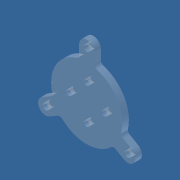
# Autodesk Inventor part: acrylic gripper plate
Saved by Autodesk Inventor 2012 (Build 160160000, 160)
## iProperties
Created: 2012-07-09
Part Number: acrylic gripper plate
Material: Polycarbonate, Clear
Document SubType Name: Modeling
Designer: Ed
Density: 1.2 g/cm^3
Mass: 25.0614 g
Surface Area: 89.5421 cm^2
Volume: 20.8845 cm^3
Author: Ed
Autodesk Inventor part; units mm, degrees
ref_plane "YZ Plane" through (0, 0, 0) normal (1, 0, 0) x (0, 1, 0)
ref_plane "XZ Plane" through (0, 0, 0) normal (0, 1, 0) x (-1, 0, 0)
ref_plane "XY Plane" through (0, 0, 0) normal (0, 0, 1) x (1, 0, 0)
sketch "Sketch1" plane through (0, 0, 0) normal (0, 0, 1) x (1, 0, 0)
  circle A0 centre (0, 0) radius 30
  line L0 (-6.35, 29.3203) -> (6.35, 29.3203)
  line L1 (6.35, 29.3203) -> (6.35, 40)
  line L2 (-6.35, 40) -> (-6.35, 29.3203)
  arc A1 (0, 46.35) -> (-6.35, 40) centre (0, 40) ccw
  arc A2 (6.35, 40) -> (0, 46.35) centre (0, 40) ccw
  line L3 (-22.2171, -20.1594) -> (-28.5671, -9.1609)
  line L4 (-28.5671, -9.1609) -> (-37.816, -14.5007)
  line L5 (-31.466, -25.4993) -> (-22.2171, -20.1594)
  arc A3 (-40.1403, -23.175) -> (-31.466, -25.4993) centre (-34.641, -20) ccw
  arc A4 (-37.816, -14.5007) -> (-40.1403, -23.175) centre (-34.641, -20) ccw
  line L6 (28.5671, -9.1609) -> (22.2171, -20.1594)
  line L7 (22.2171, -20.1594) -> (31.466, -25.4993)
  line L8 (37.816, -14.5007) -> (28.5671, -9.1609)
  arc A5 (40.1403, -23.175) -> (37.816, -14.5007) centre (34.641, -20) ccw
  arc A6 (31.466, -25.4993) -> (40.1403, -23.175) centre (34.641, -20) ccw
  point P0 (6.35, 46.35)
  point P1 (-6.35, 46.35)
  point P2 (0, 29.3203)
  point P3 (-43.3153, -17.6757)
  point P4 (-36.9653, -28.6743)
  point P5 (-25.3921, -14.6601)
  point P6 (36.9653, -28.6743)
  point P7 (43.3153, -17.6757)
  point P8 (25.3921, -14.6601)
  dimension "d0" = 60
  dimension "d6" = 12.7
  dimension "d7" = 6.35
  dimension "d8" = 40
  dimension "d11" = 360
  constraints: 18 end point, 12 point on circle, 6 centre point, 6 point on line, 2 horizontal, 2 tangent, 1 concentric, 1 midpoint, 1 parallel, 1 perpendicular, 1 vertical alignment, 73 other
  measures "d6" distance of point (6.35, 46.35) point (-6.35, 46.35)
  measures "d7" radius of A1
  measures "d8" distance of point (0, 0) A1.centre
extrude "Extrusion1" add sketch "Sketch1" along normal blind 5.588
fillet "Fillet1" radius 3.175 6 edges at (6.35, 29.3203, 2.794) (22.2171, -20.1594, 2.794) (-22.2171, -20.1594, 2.794) (28.5671, -9.1609, 2.794) (-28.5671, -9.1609, 2.794) (-6.35, 29.3203, 2.794)
hole "Hole1" at (0, 40, 5.588) direction (0, 0, -1) diameter 5.1054 end through all clearance for "Flat Head Machine Screw (82)" size "#10" standard "Ansi Unified Screw Threads"
pattern_circular "Circular Pattern1" count 3 over 360 about axis through (0, 0, 0) along (0, 0, 1) of "Hole1"
sketch "Sketch2" plane through (0, 0, 5.588) normal (0, 0, 1) x (1, 0, 0)
  arc A0 (29.1936, -6.909) -> (8.6134, 28.7369) centre (0, 0) ccw projected
  line L0 (-6.35, 31.7782) -> (-6.35, 40) projected
  line L1 (0, -15) -> (0, 15)
  line L2 (-15, 0) -> (15, 0)
  dimension "d26" = 30
  constraints: 4 end point, 2 horizontal alignment, 2 midpoint, 2 perpendicular, 2 vertical alignment, 1 coincident, 1 parallel
  measures "d26" distance of L1.start L1.end
hole "Hole2" at (0, 15, 5.588) at (15, 0, 5.588) at (0, -15, 5.588) at (-15, 0, 5.588) direction (0, 0, -1) diameter 4.4958 end through all clearance for "Flat Head Machine Screw (82)" size "#8" standard "Ansi Unified Screw Threads"
body "Solid1"
